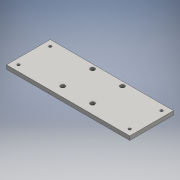
# Autodesk Inventor part: zStagePostAttach
Saved by Autodesk Inventor 2016 (Build 200138000, 138)
## iProperties
Created: 2016-09-30
Part Number: zStagePostAttach
Material: Generic
Document SubType Name: Modeling
Designer: sims01
Density: 1 g/cm^3
Appearance: Default
Author: sims01
Autodesk Inventor part; units mm, degrees
ref_plane "YZ Plane" through (0, 0, 0) normal (1, 0, 0) x (0, 1, 0)
ref_plane "XZ Plane" through (0, 0, 0) normal (0, 1, 0) x (-1, 0, 0)
ref_plane "XY Plane" through (0, 0, 0) normal (0, 0, 1) x (1, 0, 0)
sketch "Sketch1" plane through (0, 0, 0) normal (0, 0, 1) x (1, 0, 0)
  line L0 (-155, 55) -> (155, 55)
  line L1 (155, 55) -> (155, -55)
  line L2 (155, -55) -> (-155, -55)
  line L3 (-155, -55) -> (-155, 55)
  point P0 (0, 0)
  dimension "d0" = 110
  dimension "d1" = 310
  dimension "d2" = 155
  dimension "d3" = 55
  constraints: 8 end point, 2 parallel, 1 horizontal, 1 perpendicular
  measures "d0" distance of L0.end L1.end
  measures "d1" distance of L0.start L0.end
  measures "d2" distance from line of point (0, 0) L3
  measures "d3" distance from line of point (0, 0) L0
extrude "Extrusion1" add sketch "Sketch1" along normal blind 10
sketch "Sketch2" plane through (0, 0, 10) normal (0, 0, 1) x (1, 0, 0)
  line L0 (155, 55) -> (-155, 55) projected
  point P0 (0, 0)
  point P1 (-37.5, 44)
  point P2 (37.5, 44)
  point P3 (-37.5, -31)
  point P4 (37.5, -31)
  dimension "d6" = 75
  dimension "d7" = 11
  dimension "d8" = 75
  dimension "d27" = 37.5
  constraints: 2 horizontal alignment, 2 vertical alignment
  measures "d6" distance of point (37.5, 44) point (-37.5, 44)
  measures "d7" distance from line of point (37.5, 44) L0
  measures "d8" distance of point (-37.5, -31) point (-37.5, 44)
  measures "d27" horizontal distance of point (0, 0) point (37.5, 44)
hole "Hole1" at (-37.5, 44, 10) at (37.5, 44, 10) at (-37.5, -31, 10) at (37.5, -31, 10) direction (0, 0, -1) diameter 6.6 end through all counterbore diameter 11 counterbore depth 7 clearance for "Hex Head Cap Screw ISO 24017" size "M6" standard "ISO"
sketch "Sketch3" plane through (0, 0, 0) normal (0, 0, -1) x (-1, 0, 0)
  point P0 (0, 0)
  point P1 (-140, 40)
  point P2 (-140, -40)
  point P3 (140, 40)
  point P4 (140, -40)
  dimension "d16" = 80
  dimension "d17" = 40
  dimension "d18" = 280
  dimension "d19" = 140
  constraints: 2 horizontal alignment, 2 vertical alignment
  measures "d16" distance of point (-140, -40) point (-140, 40)
  measures "d17" vertical distance of point (0, 0) point (-140, 40)
  measures "d18" distance of point (140, 40) point (-140, 40)
  measures "d19" horizontal distance of point (0, 0) point (-140, 40)
hole "Hole2" at (140, 40, 0) at (140, -40, 0) at (-140, 40, 0) at (-140, -40, 0) direction (0, 0, 1) diameter 6.6 end through all counterbore diameter 11 counterbore depth 7 clearance for "Hex Head Cap Screw ISO 24017" size "M6" standard "ISO"
equation "\"d2\" = 0.5 * d1"
equation "\"d3\" = 0.5 * d0"
equation "\"d27\" = 0.5 * d6"
equation "\"d17\" = 0.5 * d16"
equation "\"d19\" = 0.5 * d18"
body "Solid1"
